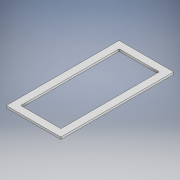
# Autodesk Inventor part: top
Saved by Autodesk Inventor 2020 (Build 240168000, 168)
## iProperties
Created: 2019-11-30
Part Number: top
Material: Générique
Document SubType Name: Modeling
Designer: bapti
Density: 1 g/cm^3
Appearance: Par défaut
Author: bapti
Autodesk Inventor part; units mm, degrees
ref_plane "YZ Plane" through (0, 0, 0) normal (1, 0, 0) x (0, 1, 0)
ref_plane "XZ Plane" through (0, 0, 0) normal (0, 1, 0) x (-1, 0, 0)
ref_plane "XY Plane" through (0, 0, 0) normal (0, 0, 1) x (1, 0, 0)
sketch "Esquisse1" plane through (0, 0, 0) normal (0, 1, 0) x (-1, 0, 0)
  line L0 (2, 0) -> (148, 0)
  line L1 (150, -2) -> (150, -308)
  line L2 (148, -310) -> (2, -310)
  line L3 (0, -308) -> (0, -2)
  line L4 (20, 0) -> (20, -20) construction
  line L5 (20, -20) -> (0, -20) construction
  line L6 (150, 0) -> (0, -310) construction
  line L7 (150, -310) -> (0, 0) construction
  line L8 (75, 0) -> (75, -310) construction
  line L9 (150, -155) -> (0, -155) construction
  line L10 (20, -20) -> (0, 0) construction
  line L11 (0, -20) -> (20, 0) construction
  line L12 (22, -20) -> (128, -20)
  line L13 (130, -22) -> (130, -288)
  line L14 (128, -290) -> (22, -290)
  line L15 (20, -288) -> (20, -22)
  line L16 (130, -290) -> (150, -290) construction
  line L17 (130, -290) -> (130, -310) construction
  arc A0 (128, -290) -> (130, -288) centre (128, -288) ccw
  arc A1 (20, -288) -> (22, -290) centre (22, -288) ccw
  arc A2 (22, -20) -> (20, -22) centre (22, -22) ccw
  arc A3 (130, -22) -> (128, -20) centre (128, -22) ccw
  arc A4 (150, -2) -> (148, 0) centre (148, -2) ccw
  arc A5 (2, 0) -> (0, -2) centre (2, -2) ccw
  arc A6 (0, -308) -> (2, -310) centre (2, -308) ccw
  arc A7 (148, -310) -> (150, -308) centre (148, -308) ccw
  dimension "d0" = 150
  dimension "d1" = 310
  dimension "d5" = 20
  dimension "d11" = 2
  constraints: 36 end point, 16 point on circle, 16 point on line, 16 tangent, 8 centre point, 8 perpendicular, 7 equal radius, 4 midpoint, 4 parallel, 2 horizontal, 1 vertical
  measures "d0" distance of L7.start L6.end
  measures "d1" distance of L6.end L7.end
  measures "d5" distance of L4.end L5.end
  measures "d11" radius of A0
extrude "Extrusion1" add sketch "Esquisse1" along normal blind 6
